Autodesk Inventor part; units mm, degrees
(part 2 of 2)
  spline S258 degree 2 poles (-59.7086, 112.4694) (-59.5777, 112.5929) (-59.1997, 112.7238) (-58.9256, 112.7238) knots 0 0 0 1 2 2 2
  line L240 (-58.9256, 112.7238) -> (-58.7156, 112.7238)
  line L241 (-58.7156, 112.7238) -> (-58.7156, 111.1405)
  spline S259 degree 2 poles (-58.7156, 111.1405) (-58.318, 111.1405) (-57.8956, 111.5407) (-57.8956, 111.8963) knots 0 0 0 1 2 2 2
  spline S260 degree 2 poles (-57.8956, 111.8963) (-57.8956, 112.0223) (-57.9524, 112.2668) (-57.9969, 112.3656) knots 0 0 0 1 2 2 2
  spline S261 degree 2 poles (-57.9969, 112.3656) (-58.0463, 112.4694) (-58.1327, 112.6126) (-58.1722, 112.6596) knots 0 0 0 1 2 2 2
  line L242 (-58.1722, 112.6596) -> (-58.1722, 112.6818)
  line L243 (-58.1722, 112.6818) -> (-57.7523, 112.6818)
  spline S262 degree 2 poles (-57.7523, 112.6818) (-57.7251, 112.6151) (-57.6461, 112.4126) (-57.6239, 112.3335) knots 0 0 0 1 2 2 2
  spline S263 degree 2 poles (-57.6239, 112.3335) (-57.5918, 112.2224) (-57.5597, 112.0396) (-57.5597, 111.9013) knots 0 0 0 1 2 2 2
  spline S264 degree 2 poles (-59.0096, 112.3484) (-59.1652, 112.3434) (-59.3924, 112.2792) (-59.469, 112.2174) knots 0 0 0 1 2 2 2
  spline S265 degree 2 poles (-59.469, 112.2174) (-59.5554, 112.1508) (-59.6468, 111.9408) (-59.6468, 111.7852) knots 0 0 0 1 2 2 2
  spline S266 degree 2 poles (-59.6468, 111.7852) (-59.6468, 111.6321) (-59.5554, 111.4172) (-59.4665, 111.3282) knots 0 0 0 1 2 2 2
  spline S267 degree 2 poles (-59.4665, 111.3282) (-59.3751, 111.2418) (-59.1553, 111.1529) (-59.0096, 111.1405) knots 0 0 0 1 2 2 2
  line L244 (-59.0096, 111.1405) -> (-59.0096, 112.3484)
  point P0 (0, 0)
  constraints: 2 other
extrude "Extrusion3" cut sketch "Sketch3" against normal blind 1
body "Solid1"
